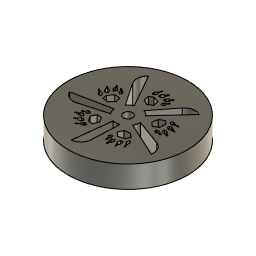
Mouse wheel (Autodesk Fusion 360 design; units mm, degrees)
Autodesk Fusion 360 part; units mm, degrees
(part 1 of 2)
sketch "Sketch1" plane through (0, 0, 0) normal (0, 0, 1) x (1, 0, 0)
  line L0 (-1.4367, 0.431) -> (1.4367, -0.431) construction
  arc A0 (-1.118, 1) -> (1.118, 1) centre (0, 0) ccw
  line L1 (-1.118, 1) -> (1.118, 1)
  line L2 (1.4367, 0.431) -> (-1.4367, -0.431) construction
  circle A1 centre (0, 0) radius 19
  dimension "d1" = 3
  dimension "d2" = 38
  constraint coincident A0.centre A1.centre
  constraint coincident L0 A0.centre
  constraint coincident A0 L2.end
  constraint coincident A0 L0.start
  constraint coincident A0 L0.end
  constraint coincident A0 L2.start
  constraint concentric A0 A1
  measures "d1" diameter of A0
  measures "d2" diameter of A1
extrude "Extrude1" add sketch "Sketch1" against normal blind 7 contours A0 L1 | A1
sketch "Sketch2" plane through (0, 0, 0) normal (0, 0, 1) x (-1, 0, 0)
  circle A0 centre (0, 0) radius 19
  circle A1 centre (0, 0) radius 3.5
  circle A2 centre (0, 0) radius 14
  dimension "d6" = 7
  dimension "d7" = 5
  constraint concentric A1 A2
  measures "d6" diameter of A1
  measures "d7" distance of A0 A2
sketch "Sketch3" plane through (0, 0, 0) normal (0, 0, 1) x (-1, 0, 0)
  line L0 (1.4245, 3.197) -> (4.8033, 7.8695)
  line L1 (4.8033, 7.8695) -> (-0.831, 15.5019)
  line L2 (-1.4884, 3.1677) -> (1.812, 7.535)
  line L3 (1.812, 7.535) -> (-5.6083, 14.6274)
  line L4 (-5.6083, 14.6274) -> (-0.831, 15.5019)
  line L5 (-1.4884, 3.1677) -> (-0.63, 3.41)
  line L6 (-0.63, 3.41) -> (1.4245, 3.197)
  line L7 (-3.4727, -0.4367) -> (-6.6062, 4.0518)
  line L8 (-2.6003, 2.3427) -> (-6, 7)
  line L9 (-6, 7) -> (-15, 4)
  line L10 (-6.6062, 4.0518) -> (-15.6446, -0.8137)
  line L11 (-15.6446, -0.8137) -> (-15, 4)
  line L12 (-3.4378, 0.4546) -> (-2.6003, 2.3427)
  line L13 (-3.4727, -0.4367) -> (-3.4378, 0.4546)
  line L14 (-0.6578, -3.4376) -> (-5.8949, -5.0308)
  line L15 (-3.0316, -1.7491) -> (-8.5115, -3.5432)
  line L16 (-8.5115, -3.5432) -> (-8.4395, -13.0298)
  line L17 (-5.8949, -5.0308) -> (-4.0605, -15.1303)
  line L18 (-4.0605, -15.1303) -> (-8.4395, -13.0298)
  line L19 (-1.4947, -3.1291) -> (-3.0316, -1.7491)
  line L20 (-0.6578, -3.4376) -> (-1.4947, -3.1291)
  line L21 (3.0661, -1.6879) -> (2.963, -7.161)
  line L22 (0.7267, -3.4237) -> (0.7396, -9.1898)
  line L23 (0.7396, -9.1898) -> (9.7841, -12.0528)
  line L24 (2.963, -7.161) -> (13.135, -8.5373)
  line L25 (13.135, -8.5373) -> (9.7841, -12.0528)
  line L26 (2.514, -2.3884) -> (0.7267, -3.4237)
  line L27 (3.0661, -1.6879) -> (2.514, -2.3884)
  line L28 (2.5528, 2.3945) -> (7.7261, 0.6051)
  line L29 (3.4807, -0.3669) -> (8.9686, -2.1364)
  line L30 (8.9686, -2.1364) -> (14.4864, 5.5807)
  line L31 (7.7261, 0.6051) -> (12.1784, 9.854)
  line L32 (12.1784, 9.854) -> (14.4864, 5.5807)
  line L33 (3.0484, 1.6529) -> (3.4807, -0.3669)
  line L34 (2.5528, 2.3945) -> (3.0484, 1.6529)
  circle A0 centre (0, 0) radius 19
  dimension "d11" = 360
sketch "Sketch4" plane through (0, 0, 0) normal (0, 0, 1) x (-1, 0, 0)
  circle A0 centre (0, 0) radius 19
  circle A1 centre (0, 0) radius 1.45
  dimension "d30" = 2.9
  constraint coincident A0.centre A1.centre
  measures "d30" diameter of A1
sketch "Sketch6" plane through (0, 0, 0) normal (0, 0, 1) x (-1, 0, 0)
  circle A0 centre (0, 0) radius 19
sketch "Sketch7" plane through (0, 0, 0) normal (0, 0, 1) x (-1, 0, 0)
  line L0 (0, -6) -> (1.6404, -6.8063)
  line L1 (1.6404, -6.8063) -> (2, -8.5)
  line L2 (2, -8.5) -> (0.8202, -9.1077)
  line L3 (0.8202, -9.1077) -> (-1, -8.5)
  line L4 (-1, -8.5) -> (-1.357, -6.8189)
  line L5 (-1.357, -6.8189) -> (0, -6)
  line L6 (1.9455, -9.6677) -> (2.2324, -10.2247)
  line L7 (2.2324, -10.2247) -> (2.0889, -10.6544)
  line L8 (2.0889, -10.6544) -> (1.4101, -11.4226)
  line L9 (1.4101, -11.4226) -> (1.2014, -10.4396)
  line L10 (1.2014, -10.4396) -> (1.3057, -10.127)
  line L11 (1.3057, -10.127) -> (1.9455, -9.6677)
  line L12 (0.4215, -10.1911) -> (0.4215, -10.8376)
  line L13 (0.4215, -10.8376) -> (-0.1481, -11.4996)
  line L14 (-0.1481, -11.4996) -> (-0.7484, -11.4996)
  line L15 (-0.7484, -11.4996) -> (-0.7484, -10.5143)
  line L16 (-0.7484, -10.5143) -> (-0.1481, -10.0371)
  line L17 (-0.1481, -10.0371) -> (0.4215, -10.1911)
  line L18 (-1.3334, -9.8678) -> (-1.5082, -10.5143)
  line L19 (-1.5082, -10.5143) -> (-2.1168, -10.9982)
  line L20 (-2.1168, -10.9982) -> (-2.5, -10.9982)
  line L21 (-2.5, -10.9982) -> (-2.7496, -10.5143)
  line L22 (-2.7496, -10.5143) -> (-2.3084, -9.7293)
  line L23 (-2.3084, -9.7293) -> (-1.3334, -9.8678)
  line L24 (-2.3084, -9.1135) -> (-3.0575, -9.2674)
  line L25 (-3.0575, -9.2674) -> (-3.1911, -8.6176)
  line L26 (-2.3084, -9.1135) -> (-2.1907, -8.2851)
  line L27 (-2.1907, -8.2851) -> (-2.8295, -8.1943)
  line L28 (-2.8295, -8.1943) -> (-3.1911, -8.6176)
  line L29 (1.4529, -11.869) -> (1.1049, -12.2764)
  line L30 (1.1049, -12.2764) -> (1.1894, -11.6818)
  line L31 (1.1894, -11.6818) -> (1.4101, -11.6349)
  line L32 (1.4101, -11.6349) -> (1.4529, -11.869)
  line L33 (-0.5833, -11.869) -> (-0.9521, -12.3007)
  line L34 (-0.9521, -12.3007) -> (-0.9521, -11.7519)
  line L35 (-0.9521, -11.7519) -> (-0.7677, -11.7519)
  line L36 (-0.7677, -11.7519) -> (-0.5833, -11.869)
  line L37 (-2.6562, -11.3012) -> (-3.1065, -11.6591)
  line L38 (-3.1065, -11.6591) -> (-2.9735, -11.007)
  line L39 (-2.9735, -11.007) -> (-2.7469, -11.007)
  line L40 (-2.7469, -11.007) -> (-2.6562, -11.3012)
  line L41 (-3.04, -9.5445) -> (-3.04, -9.7825)
  line L42 (-3.04, -9.7825) -> (-3.4222, -10.0863)
  line L43 (-3.4222, -10.0863) -> (-3.4222, -9.6635)
  line L44 (-3.4222, -9.6635) -> (-3.2311, -9.5116)
  line L45 (-3.2311, -9.5116) -> (-3.04, -9.5445)
  line L46 (11.2993, -2.1887) -> (10.2999, -2.0834)
  line L47 (10.7785, -1.3057) -> (11.2993, -2.1887)
  line L48 (10.4141, -1.0365) -> (10.7785, -1.3057)
  line L49 (9.7957, -1.1372) -> (10.4141, -1.0365)
  line L50 (10.0348, -1.8876) -> (9.7957, -1.1372)
  line L51 (10.2999, -2.0834) -> (10.0348, -1.8876)
  line L52 (8.702, -0.7245) -> (8.9154, -2.0344)
  line L53 (6.9801, -0.5432) -> (8.702, -0.7245)
  line L54 (5.7063, -1.8541) -> (6.9801, -0.5432)
  line L55 (6.0658, -3.3977) -> (5.7063, -1.8541)
  line L56 (7.775, -3.5777) -> (6.0658, -3.3977)
  line L57 (8.9154, -2.0344) -> (7.775, -3.5777)
  line L58 (7.2026, -4.6437) -> (6.9189, -5.2232)
  line L59 (7.9541, -5.0117) -> (7.2026, -4.6437)
  line L60 (7.9541, -5.0117) -> (7.869, -5.7717)
  line L61 (7.869, -5.7717) -> (7.2097, -5.6979)
  line L62 (6.9189, -5.2232) -> (7.2097, -5.6979)
  line L63 (10.4374, -2.9482) -> (10.891, -3.6944)
  line L64 (9.8225, -2.7484) -> (10.4374, -2.9482)
  line L65 (9.5001, -3.2425) -> (9.8225, -2.7484)
  line L66 (9.7685, -3.9609) -> (9.5001, -3.2425)
  line L67 (10.7054, -4.2654) -> (9.7685, -3.9609)
  line L68 (10.891, -3.6944) -> (10.7054, -4.2654)
  line L69 (12.0169, -2.7428) -> (11.4775, -2.4787)
  line L70 (11.7371, -2.286) -> (12.0169, -2.7428)
  line L71 (11.5012, -2.2543) -> (11.7371, -2.286)
  line L72 (11.4775, -2.4787) -> (11.5012, -2.2543)
  line L73 (11.1078, -4.2225) -> (11.4045, -4.7067)
  line L74 (10.9395, -4.3617) -> (11.1078, -4.2225)
  line L75 (10.8825, -4.5371) -> (10.9395, -4.3617)
  line L76 (11.4045, -4.7067) -> (10.8825, -4.5371)
  line L77 (9.5337, -4.6835) -> (9.8057, -5.4118)
  line L78 (8.9728, -4.3175) -> (9.5337, -4.6835)
  line L79 (8.5397, -5.2019) -> (8.9728, -4.3175)
  line L80 (9.1501, -5.8642) -> (8.5397, -5.2019)
  line L81 (9.6873, -5.7763) -> (9.1501, -5.8642)
  line L82 (9.8057, -5.4118) -> (9.6873, -5.7763)
  line L83 (9.9272, -6.0184) -> (10.1285, -6.5574)
  line L84 (9.6194, -6.0137) -> (9.9272, -6.0184)
  line L85 (10.1285, -6.5574) -> (9.5494, -6.2293)
  line L86 (9.5494, -6.2293) -> (9.6194, -6.0137)
  line L87 (8.3643, -5.9142) -> (8.5351, -6.3715)
  line L88 (8.5351, -6.3715) -> (8.133, -6.2409)
  line L89 (8.133, -6.2409) -> (8.0476, -6.0122)
  line L90 (8.0476, -6.0122) -> (8.138, -5.8407)
  line L91 (8.138, -5.8407) -> (8.3643, -5.9142)
  line L92 (5.5732, 10.0699) -> (5.1643, 9.1519)
  line L93 (4.5725, 9.8475) -> (5.5732, 10.0699)
  line L94 (4.2039, 9.5842) -> (4.5725, 9.8475)
  line L95 (4.1086, 8.9648) -> (4.2039, 9.5842)
  line L96 (4.8961, 8.9604) -> (4.1086, 8.9648)
  line L97 (5.1643, 9.1519) -> (4.8961, 8.9604)
  line L98 (3.3781, 8.0522) -> (4.6898, 7.8504)
  line L99 (2.6736, 6.4706) -> (3.3781, 8.0522)
  line L100 (3.5267, 4.8541) -> (2.6736, 6.4706)
  line L101 (5.1059, 4.719) -> (3.5267, 4.8541)
  line L102 (5.8052, 6.2889) -> (5.1059, 4.719)
  line L103 (4.6898, 7.8504) -> (5.8052, 6.2889)
  line L104 (6.6422, 5.4151) -> (7.1056, 4.9662)
  line L105 (7.2243, 6.0161) -> (6.6422, 5.4151)
  line L106 (7.2243, 6.0161) -> (7.9209, 5.7004)
  line L107 (7.9209, 5.7004) -> (7.6469, 5.0961)
  line L108 (7.1056, 4.9662) -> (7.6469, 5.0961)
  line L109 (6.0292, 9.0156) -> (6.8791, 9.2163)
  line L110 (5.6492, 8.4925) -> (6.0292, 9.0156)
  line L111 (6.0195, 8.0332) -> (5.6492, 8.4925)
  line L112 (6.7857, 8.0664) -> (6.0195, 8.0332)
  line L113 (7.3648, 8.8634) -> (6.7857, 8.0664)
  line L114 (6.8791, 9.2163) -> (7.3648, 8.8634)
  line L115 (6.322, 10.5812) -> (5.9041, 10.1498)
  line L116 (5.801, 10.4562) -> (6.322, 10.5812)
  line L117 (5.698, 10.2417) -> (5.801, 10.4562)
  line L118 (5.9041, 10.1498) -> (5.698, 10.2417)
  line L119 (7.4483, 9.2594) -> (8.0005, 9.3919)
  line L120 (7.5287, 9.0563) -> (7.4483, 9.2594)
  line L121 (7.6779, 8.9479) -> (7.5287, 9.0563)
  line L122 (8.0005, 9.3919) -> (7.6779, 8.9479)
  line L123 (7.4003, 7.6198) -> (8.1771, 7.6535)
  line L124 (6.8789, 7.1995) -> (7.4003, 7.6198)
  line L125 (7.5863, 6.5143) -> (6.8789, 7.1995)
  line L126 (8.4047, 6.8901) -> (7.5863, 6.5143)
  line L127 (8.4871, 7.4282) -> (8.4047, 6.8901)
  line L128 (8.1771, 7.6535) -> (8.4871, 7.4282)
  line L129 (8.7916, 7.5816) -> (9.3663, 7.6065)
  line L130 (8.692, 7.2903) -> (8.7916, 7.5816)
  line L131 (9.3663, 7.6065) -> (8.8753, 7.157)
  line L132 (8.8753, 7.157) -> (8.692, 7.2903)
  line L133 (8.2095, 6.1273) -> (8.6972, 6.1485)
  line L134 (8.6972, 6.1485) -> (8.4487, 5.8064)
  line L135 (8.4487, 5.8064) -> (8.2048, 5.7959)
  line L136 (8.2048, 5.7959) -> (8.0696, 5.9348)
  line L137 (8.0696, 5.9348) -> (8.2095, 6.1273)
  line L138 (-7.8548, 8.4122) -> (-7.1081, 7.7396)
  line L139 (-7.9525, 7.3918) -> (-7.8548, 8.4122)
  line L140 (-7.816, 6.9598) -> (-7.9525, 7.3918)
  line L141 (-7.2564, 6.6778) -> (-7.816, 6.9598)
  line L142 (-7.0089, 7.4254) -> (-7.2564, 6.6778)
  line L143 (-7.1081, 7.7396) -> (-7.0089, 7.4254)
  line L144 (-6.6142, 5.7011) -> (-6.0169, 6.8862)
  line L145 (-5.3277, 4.5422) -> (-6.6142, 5.7011)
  line L146 (-3.5267, 4.8541) -> (-5.3277, 4.5422)
  line L147 (-2.9103, 6.3142) -> (-3.5267, 4.8541)
  line L148 (-4.1872, 7.4644) -> (-2.9103, 6.3142)
  line L149 (-6.0169, 6.8862) -> (-4.1872, 7.4644)
  line L150 (-3.0976, 7.9904) -> (-2.5274, 8.2925)
  line L151 (-3.4892, 8.7298) -> (-3.0976, 7.9904)
  line L152 (-3.4892, 8.7298) -> (-2.9737, 9.2947)
  line L153 (-2.9737, 9.2947) -> (-2.4836, 8.8474)
  line L154 (-2.5274, 8.2925) -> (-2.4836, 8.8474)
  line L155 (-6.7112, 8.5201) -> (-6.6395, 9.3904)
  line L156 (-6.3312, 7.997) -> (-6.7112, 8.5201)
  line L157 (-5.7799, 8.2073) -> (-6.3312, 7.997)
  line L158 (-5.5747, 8.9462) -> (-5.7799, 8.2073)
  line L159 (-6.1538, 9.7433) -> (-5.5747, 8.9462)
  line L160 (-6.6395, 9.3904) -> (-6.1538, 9.7433)
  line L161 (-8.1097, 9.2824) -> (-7.8286, 8.7516)
  line L162 (-8.1518, 8.7483) -> (-8.1097, 9.2824)
  line L163 (-7.9796, 8.584) -> (-8.1518, 8.7483)
  line L164 (-7.8286, 8.7516) -> (-7.9796, 8.584)
  line L165 (-6.5045, 9.9451) -> (-6.4599, 10.5111)
  line L166 (-6.2865, 9.9588) -> (-6.5045, 9.9451)
  line L167 (-6.1373, 10.0672) -> (-6.2865, 9.9588)
  line L168 (-6.4599, 10.5111) -> (-6.1373, 10.0672)
  line L169 (-4.9601, 9.3928) -> (-4.752, 10.1419)
  line L170 (-4.7214, 8.767) -> (-4.9601, 9.3928)
  line L171 (-3.8512, 9.228) -> (-4.7214, 8.767)
  line L172 (-3.9557, 10.1225) -> (-3.8512, 9.228)
  line L173 (-4.442, 10.3672) -> (-3.9557, 10.1225)
  line L174 (-4.752, 10.1419) -> (-4.442, 10.3672)
  line L175 (-4.4938, 10.7041) -> (-4.3398, 11.2584)
  line L176 (-4.2475, 10.5194) -> (-4.4938, 10.7041)
  line L177 (-4.3398, 11.2584) -> (-4.0641, 10.6526)
  line L178 (-4.0641, 10.6526) -> (-4.2475, 10.5194)
  line L179 (-3.2906, 9.7011) -> (-3.16, 10.1715)
  line L180 (-3.16, 10.1715) -> (-2.9115, 9.8295)
  line L181 (-2.9115, 9.8295) -> (-2.9768, 9.5943)
  line L182 (-2.9768, 9.5943) -> (-3.1507, 9.5086)
  line L183 (-3.1507, 9.5086) -> (-3.2906, 9.7011)
  line L184 (-10.4278, -4.8709) -> (-9.5574, -4.3686)
  line L185 (-9.4874, -5.2791) -> (-10.4278, -4.8709)
  line L186 (-9.0344, -5.2828) -> (-9.4874, -5.2791)
  line L187 (-8.5933, -4.8377) -> (-9.0344, -5.2828)
  line L188 (-9.2278, -4.3712) -> (-8.5933, -4.8377)
  line L189 (-9.5574, -4.3686) -> (-9.2278, -4.3712)
  line L190 (-7.4659, -4.5288) -> (-8.4085, -3.5945)
  line L191 (-5.9663, -3.6633) -> (-7.4659, -4.5288)
  line L192 (-5.7063, -1.8541) -> (-5.9663, -3.6633)
  line L193 (-6.9045, -0.8166) -> (-5.7063, -1.8541)
  line L194 (-8.393, -1.6756) -> (-6.9045, -0.8166)
  line L195 (-8.4085, -3.5945) -> (-8.393, -1.6756)
  line L196 (-8.5566, -0.4768) -> (-8.6676, 0.1588)
  line L197 (-9.3808, -0.6208) -> (-8.5566, -0.4768)
  line L198 (-9.3808, -0.6208) -> (-9.7587, 0.0441)
  line L199 (-9.7587, 0.0441) -> (-9.1819, 0.3719)
  line L200 (-8.6676, 0.1588) -> (-9.1819, 0.3719)
  line L201 (-10.1769, -3.7499) -> (-10.9825, -3.4127)
  line L202 (-9.562, -3.5501) -> (-10.1769, -3.7499)
  line L203 (-9.5916, -2.9608) -> (-9.562, -3.5501)
  line L204 (-10.231, -2.5373) -> (-9.5916, -2.9608)
  line L205 (-11.168, -2.8417) -> (-10.231, -2.5373)
  line L206 (-10.9825, -3.4127) -> (-11.168, -2.8417)
  line L207 (-11.3341, -4.8444) -> (-10.7425, -4.741)
  line L208 (-10.8391, -5.0495) -> (-11.3341, -4.8444)
  line L209 (-10.6297, -4.9365) -> (-10.8391, -5.0495)
  line L210 (-10.7425, -4.741) -> (-10.6297, -4.9365)
  line L211 (-11.4683, -3.113) -> (-11.9929, -2.8956)
  line L212 (-11.414, -2.9014) -> (-11.4683, -3.113)
  line L213 (-11.471, -2.726) -> (-11.414, -2.9014)
  line L214 (-11.9929, -2.8956) -> (-11.471, -2.726)
  line L215 (-10.4658, -1.8148) -> (-11.114, -1.3854)
  line L216 (-9.7969, -1.7812) -> (-10.4658, -1.8148)
  line L217 (-9.9664, -0.8111) -> (-9.7969, -1.7812)
  line L218 (-10.8494, -0.634) -> (-9.9664, -0.8111)
  line L219 (-11.2324, -1.021) -> (-10.8494, -0.634)
  line L220 (-11.114, -1.3854) -> (-11.2324, -1.021)
  line L221 (-11.5688, -0.9661) -> (-12.0485, -0.6484)
  line L222 (-11.3171, -0.7889) -> (-11.5688, -0.9661)
  line L223 (-12.0485, -0.6484) -> (-11.3871, -0.5734)
  line L224 (-11.3871, -0.5734) -> (-11.3171, -0.7889)
  line L225 (-10.2432, -0.1317) -> (-10.6502, 0.1379)
  line L226 (-10.6502, 0.1379) -> (-10.2481, 0.2685)
  line L227 (-10.2481, 0.2685) -> (-10.0446, 0.1337)
  line L228 (-10.0446, 0.1337) -> (-10.0168, -0.0582)
  line L229 (-10.0168, -0.0582) -> (-10.2432, -0.1317)
  dimension "d34" = 360
  constraint parallel L1 L4
  constraint perpendicular L2 L6
  constraint perpendicular L3 L7
  constraint parallel L4 L9
  constraint perpendicular L3 L10
  constraint vertical L12
  constraint horizontal L14
  constraint perpendicular L14 L15
  constraint perpendicular L17 L18
  constraint parallel L16 L19
  constraint perpendicular L12 L20
  constraint perpendicular L24 L25
  constraint perpendicular L23 L26
  constraint perpendicular L26 L27
  constraint parallel L28 L29
  constraint perpendicular L23 L30
  constraint perpendicular L9 L31
  constraint parallel L29 L33
  constraint vertical L34
  constraint perpendicular L34 L35
  constraint parallel L16 L37
  constraint perpendicular L39 L41
  constraint parallel L37 L42
  constraint perpendicular L39 L43
  constraint parallel L37 L44
extrude "Extrude9" cut sketch "Sketch7" against normal blind 17
sketch "Sketch8" plane through (0, 0, 0) normal (0, 0, 1) x (-1, 0, 0)
  line L0 (-3.1065, -11.6591) -> (-2.9735, -11.007)
  line L1 (-2.9735, -11.007) -> (-2.7469, -11.007)
  line L2 (-2.7469, -11.007) -> (-2.6562, -11.3012)
  line L3 (-2.6562, -11.3012) -> (-3.1065, -11.6591)
  line L4 (-11.5688, -0.9661) -> (-12.0485, -0.6484)
  line L5 (-12.0485, -0.6484) -> (-11.3871, -0.5734)
  line L6 (-11.3871, -0.5734) -> (-11.3171, -0.7889)
  line L7 (-11.3171, -0.7889) -> (-11.5688, -0.9661)
  line L8 (-4.4938, 10.7041) -> (-4.3398, 11.2584)
  line L9 (-4.3398, 11.2584) -> (-4.0641, 10.6526)
  line L10 (-4.0641, 10.6526) -> (-4.2475, 10.5194)
  line L11 (-4.2475, 10.5194) -> (-4.4938, 10.7041)
  line L12 (8.7916, 7.5816) -> (9.3663, 7.6065)
  line L13 (9.3663, 7.6065) -> (8.8753, 7.157)
  line L14 (8.8753, 7.157) -> (8.692, 7.2903)
  line L15 (8.692, 7.2903) -> (8.7916, 7.5816)
  line L16 (9.9272, -6.0184) -> (10.1285, -6.5574)
  line L17 (10.1285, -6.5574) -> (9.5494, -6.2293)
  line L18 (9.5494, -6.2293) -> (9.6194, -6.0137)
  line L19 (9.6194, -6.0137) -> (9.9272, -6.0184)
  line L20 (-2.5, -10.9982) -> (-2.7496, -10.5143)
  line L21 (-2.7496, -10.5143) -> (-2.3084, -9.7293)
  line L22 (-2.3084, -9.7293) -> (-1.3334, -9.8678)
  line L23 (-1.3334, -9.8678) -> (-1.5082, -10.5143)
  line L24 (-1.5082, -10.5143) -> (-2.1168, -10.9982)
  line L25 (-2.1168, -10.9982) -> (-2.5, -10.9982)
  line L26 (-9.7969, -1.7812) -> (-10.4658, -1.8148)
  line L27 (-10.4658, -1.8148) -> (-11.114, -1.3854)
  line L28 (-11.114, -1.3854) -> (-11.2324, -1.021)
  line L29 (-11.2324, -1.021) -> (-10.8494, -0.634)
  line L30 (-10.8494, -0.634) -> (-9.9664, -0.8111)
  line L31 (-9.9664, -0.8111) -> (-9.7969, -1.7812)
  line L32 (-4.7214, 8.767) -> (-4.9601, 9.3928)
  line L33 (-4.9601, 9.3928) -> (-4.752, 10.1419)
  line L34 (-4.752, 10.1419) -> (-4.442, 10.3672)
  line L35 (-4.442, 10.3672) -> (-3.9557, 10.1225)
  line L36 (-3.9557, 10.1225) -> (-3.8512, 9.228)
  line L37 (-3.8512, 9.228) -> (-4.7214, 8.767)
  line L38 (6.8789, 7.1995) -> (7.4003, 7.6198)
  line L39 (7.4003, 7.6198) -> (8.1771, 7.6535)
  line L40 (8.1771, 7.6535) -> (8.4871, 7.4282)
  line L41 (8.4871, 7.4282) -> (8.4047, 6.8901)
  line L42 (8.4047, 6.8901) -> (7.5863, 6.5143)
  line L43 (7.5863, 6.5143) -> (6.8789, 7.1995)
  line L44 (8.9728, -4.3175) -> (9.5337, -4.6835)
  line L45 (9.5337, -4.6835) -> (9.8057, -5.4118)
  line L46 (9.8057, -5.4118) -> (9.6873, -5.7763)
  line L47 (9.6873, -5.7763) -> (9.1501, -5.8642)
  line L48 (9.1501, -5.8642) -> (8.5397, -5.2019)
  line L49 (8.5397, -5.2019) -> (8.9728, -4.3175)
  line L50 (-5.9663, -3.6633) -> (-7.4659, -4.5288)
  line L51 (-7.4659, -4.5288) -> (-8.4085, -3.5945)
  line L52 (-8.4085, -3.5945) -> (-8.393, -1.6756)
  line L53 (-8.393, -1.6756) -> (-6.9045, -0.8166)
  line L54 (-6.9045, -0.8166) -> (-5.7063, -1.8541)
  line L55 (-5.7063, -1.8541) -> (-5.9663, -3.6633)
  line L56 (-5.3277, 4.5422) -> (-6.6142, 5.7011)
  line L57 (-6.6142, 5.7011) -> (-6.0169, 6.8862)
  line L58 (-6.0169, 6.8862) -> (-4.1872, 7.4644)
  line L59 (-4.1872, 7.4644) -> (-2.9103, 6.3142)
  line L60 (-2.9103, 6.3142) -> (-3.5267, 4.8541)
  line L61 (-3.5267, 4.8541) -> (-5.3277, 4.5422)
  line L62 (6.9189, -5.2232) -> (7.2026, -4.6437)
  line L63 (7.2026, -4.6437) -> (7.9541, -5.0117)
  line L64 (7.9541, -5.0117) -> (7.869, -5.7717)
  line L65 (7.869, -5.7717) -> (7.2097, -5.6979)
  line L66 (7.2097, -5.6979) -> (6.9189, -5.2232)
  line L67 (7.1056, 4.9662) -> (6.6422, 5.4151)
  line L68 (6.6422, 5.4151) -> (7.2243, 6.0161)
  line L69 (7.2243, 6.0161) -> (7.9209, 5.7004)
  line L70 (7.9209, 5.7004) -> (7.6469, 5.0961)
  line L71 (7.6469, 5.0961) -> (7.1056, 4.9662)
  line L72 (-2.5274, 8.2925) -> (-3.0976, 7.9904)
  line L73 (-3.0976, 7.9904) -> (-3.4892, 8.7298)
  line L74 (-3.4892, 8.7298) -> (-2.9737, 9.2947)
  line L75 (-2.9737, 9.2947) -> (-2.4836, 8.8474)
  line L76 (-2.4836, 8.8474) -> (-2.5274, 8.2925)
  line L77 (-8.6676, 0.1588) -> (-8.5566, -0.4768)
  line L78 (-8.5566, -0.4768) -> (-9.3808, -0.6208)
  line L79 (-9.3808, -0.6208) -> (-9.7587, 0.0441)
  line L80 (-9.7587, 0.0441) -> (-9.1819, 0.3719)
  line L81 (-9.1819, 0.3719) -> (-8.6676, 0.1588)
  line L82 (-2.8295, -8.1943) -> (-2.1907, -8.2851)
  line L83 (-2.1907, -8.2851) -> (-2.3084, -9.1135)
  line L84 (-2.3084, -9.1135) -> (-3.0575, -9.2674)
  line L85 (-3.0575, -9.2674) -> (-3.1911, -8.6176)
  line L86 (-3.1911, -8.6176) -> (-2.8295, -8.1943)
  line L87 (8.133, -6.2409) -> (8.0476, -6.0122)
  line L88 (8.0476, -6.0122) -> (8.138, -5.8407)
  line L89 (8.138, -5.8407) -> (8.3643, -5.9142)
  line L90 (8.3643, -5.9142) -> (8.5351, -6.3715)
  line L91 (8.5351, -6.3715) -> (8.133, -6.2409)
  line L92 (8.4487, 5.8064) -> (8.2048, 5.7959)
  line L93 (8.2048, 5.7959) -> (8.0696, 5.9348)
  line L94 (8.0696, 5.9348) -> (8.2095, 6.1273)
  line L95 (8.2095, 6.1273) -> (8.6972, 6.1485)
  line L96 (8.6972, 6.1485) -> (8.4487, 5.8064)
  line L97 (-2.9115, 9.8295) -> (-2.9768, 9.5943)
  line L98 (-2.9768, 9.5943) -> (-3.1507, 9.5086)
  line L99 (-3.1507, 9.5086) -> (-3.2906, 9.7011)
  line L100 (-3.2906, 9.7011) -> (-3.16, 10.1715)
  line L101 (-3.16, 10.1715) -> (-2.9115, 9.8295)
  line L102 (-10.2481, 0.2685) -> (-10.0446, 0.1337)
  line L103 (-10.0446, 0.1337) -> (-10.0168, -0.0582)
  line L104 (-10.0168, -0.0582) -> (-10.2432, -0.1317)
  line L105 (-10.2432, -0.1317) -> (-10.6502, 0.1379)
  line L106 (-10.6502, 0.1379) -> (-10.2481, 0.2685)
  line L107 (-3.4222, -10.0863) -> (-3.4222, -9.6635)
  line L108 (-3.4222, -9.6635) -> (-3.2311, -9.5116)
  line L109 (-3.2311, -9.5116) -> (-3.04, -9.5445)
  line L110 (-3.04, -9.5445) -> (-3.04, -9.7825)
  line L111 (-3.04, -9.7825) -> (-3.4222, -10.0863)
  line L112 (-0.9521, -12.3007) -> (-0.9521, -11.7519)
  line L113 (-0.9521, -11.7519) -> (-0.7677, -11.7519)
  line L114 (-0.7677, -11.7519) -> (-0.5833, -11.869)
  line L115 (-0.5833, -11.869) -> (-0.9521, -12.3007)
  line L116 (-11.414, -2.9014) -> (-11.4683, -3.113)
  line L117 (-11.4683, -3.113) -> (-11.9929, -2.8956)
  line L118 (-11.9929, -2.8956) -> (-11.471, -2.726)
  line L119 (-11.471, -2.726) -> (-11.414, -2.9014)
  line L120 (-6.2865, 9.9588) -> (-6.5045, 9.9451)
  line L121 (-6.5045, 9.9451) -> (-6.4599, 10.5111)
  line L122 (-6.4599, 10.5111) -> (-6.1373, 10.0672)
  line L123 (-6.1373, 10.0672) -> (-6.2865, 9.9588)
  line L124 (7.5287, 9.0563) -> (7.4483, 9.2594)
  line L125 (7.4483, 9.2594) -> (8.0005, 9.3919)
  line L126 (8.0005, 9.3919) -> (7.6779, 8.9479)
  line L127 (7.6779, 8.9479) -> (7.5287, 9.0563)
  line L128 (10.9395, -4.3617) -> (11.1078, -4.2225)
  line L129 (11.1078, -4.2225) -> (11.4045, -4.7067)
  line L130 (11.4045, -4.7067) -> (10.8825, -4.5371)
  line L131 (10.8825, -4.5371) -> (10.9395, -4.3617)
  line L132 (-0.7484, -11.4996) -> (-0.7484, -10.5143)
  line L133 (-0.7484, -10.5143) -> (-0.1481, -10.0371)
  line L134 (-0.1481, -10.0371) -> (0.4215, -10.1911)
  line L135 (0.4215, -10.1911) -> (0.4215, -10.8376)
  line L136 (0.4215, -10.8376) -> (-0.1481, -11.4996)
  line L137 (-0.1481, -11.4996) -> (-0.7484, -11.4996)
  line L138 (-9.562, -3.5501) -> (-10.1769, -3.7499)
  line L139 (-10.1769, -3.7499) -> (-10.9825, -3.4127)
  line L140 (-10.9825, -3.4127) -> (-11.168, -2.8417)
  line L141 (-11.168, -2.8417) -> (-10.231, -2.5373)
  line L142 (-10.231, -2.5373) -> (-9.5916, -2.9608)
  line L143 (-9.5916, -2.9608) -> (-9.562, -3.5501)
  line L144 (-6.3312, 7.997) -> (-6.7112, 8.5201)
  line L145 (-6.7112, 8.5201) -> (-6.6395, 9.3904)
  line L146 (-6.6395, 9.3904) -> (-6.1538, 9.7433)
  line L147 (-6.1538, 9.7433) -> (-5.5747, 8.9462)
  line L148 (-5.5747, 8.9462) -> (-5.7799, 8.2073)
  line L149 (-5.7799, 8.2073) -> (-6.3312, 7.997)
  line L150 (5.6492, 8.4925) -> (6.0292, 9.0156)
  line L151 (6.0292, 9.0156) -> (6.8791, 9.2163)
  line L152 (6.8791, 9.2163) -> (7.3648, 8.8634)
  line L153 (7.3648, 8.8634) -> (6.7857, 8.0664)
  line L154 (6.7857, 8.0664) -> (6.0195, 8.0332)
  line L155 (6.0195, 8.0332) -> (5.6492, 8.4925)
  line L156 (9.8225, -2.7484) -> (10.4374, -2.9482)
  line L157 (10.4374, -2.9482) -> (10.891, -3.6944)
  line L158 (10.891, -3.6944) -> (10.7054, -4.2654)
  line L159 (10.7054, -4.2654) -> (9.7685, -3.9609)
  line L160 (9.7685, -3.9609) -> (9.5001, -3.2425)
  line L161 (9.5001, -3.2425) -> (9.8225, -2.7484)
  line L162 (0.8202, -9.1077) -> (-1, -8.5)
  line L163 (-1, -8.5) -> (-1.357, -6.8189)
  line L164 (-1.357, -6.8189) -> (0, -6)
  line L165 (0, -6) -> (1.6404, -6.8063)
  line L166 (1.6404, -6.8063) -> (2, -8.5)
  line L167 (2, -8.5) -> (0.8202, -9.1077)
  line L168 (2.6736, 6.4706) -> (3.3781, 8.0522)
  line L169 (3.3781, 8.0522) -> (4.6898, 7.8504)
  line L170 (4.6898, 7.8504) -> (5.8052, 6.2889)
  line L171 (5.8052, 6.2889) -> (5.1059, 4.719)
  line L172 (5.1059, 4.719) -> (3.5267, 4.8541)
  line L173 (3.5267, 4.8541) -> (2.6736, 6.4706)
  line L174 (6.9801, -0.5432) -> (8.702, -0.7245)
  line L175 (8.702, -0.7245) -> (8.9154, -2.0344)
  line L176 (8.9154, -2.0344) -> (7.775, -3.5777)
  line L177 (7.775, -3.5777) -> (6.0658, -3.3977)
  line L178 (6.0658, -3.3977) -> (5.7063, -1.8541)
  line L179 (5.7063, -1.8541) -> (6.9801, -0.5432)
  line L180 (10.7785, -1.3057) -> (11.2993, -2.1887)
  line L181 (11.2993, -2.1887) -> (10.2999, -2.0834)
  line L182 (10.2999, -2.0834) -> (10.0348, -1.8876)
  line L183 (10.0348, -1.8876) -> (9.7957, -1.1372)
  line L184 (9.7957, -1.1372) -> (10.4141, -1.0365)
  line L185 (10.4141, -1.0365) -> (10.7785, -1.3057)
  line L186 (4.5725, 9.8475) -> (5.5732, 10.0699)
  line L187 (5.5732, 10.0699) -> (5.1643, 9.1519)
  line L188 (5.1643, 9.1519) -> (4.8961, 8.9604)
  line L189 (4.8961, 8.9604) -> (4.1086, 8.9648)
  line L190 (4.1086, 8.9648) -> (4.2039, 9.5842)
  line L191 (4.2039, 9.5842) -> (4.5725, 9.8475)
  line L192 (-7.9525, 7.3918) -> (-7.8548, 8.4122)
  line L193 (-7.8548, 8.4122) -> (-7.1081, 7.7396)
  line L194 (-7.1081, 7.7396) -> (-7.0089, 7.4254)
  line L195 (-7.0089, 7.4254) -> (-7.2564, 6.6778)
  line L196 (-7.2564, 6.6778) -> (-7.816, 6.9598)
  line L197 (-7.816, 6.9598) -> (-7.9525, 7.3918)
  line L198 (-9.4874, -5.2791) -> (-10.4278, -4.8709)
  line L199 (-10.4278, -4.8709) -> (-9.5574, -4.3686)
  line L200 (-9.5574, -4.3686) -> (-9.2278, -4.3712)
  line L201 (-9.2278, -4.3712) -> (-8.5933, -4.8377)
  line L202 (-8.5933, -4.8377) -> (-9.0344, -5.2828)
  line L203 (-9.0344, -5.2828) -> (-9.4874, -5.2791)
  line L204 (1.4101, -11.4226) -> (1.2014, -10.4396)
  line L205 (1.2014, -10.4396) -> (1.3057, -10.127)
  line L206 (1.3057, -10.127) -> (1.9455, -9.6677)
  line L207 (1.9455, -9.6677) -> (2.2324, -10.2247)
  line L208 (2.2324, -10.2247) -> (2.0889, -10.6544)
  line L209 (2.0889, -10.6544) -> (1.4101, -11.4226)
  line L210 (11.7371, -2.286) -> (12.0169, -2.7428)
  line L211 (12.0169, -2.7428) -> (11.4775, -2.4787)
  line L212 (11.4775, -2.4787) -> (11.5012, -2.2543)
  line L213 (11.5012, -2.2543) -> (11.7371, -2.286)
  line L214 (5.801, 10.4562) -> (6.322, 10.5812)
  line L215 (6.322, 10.5812) -> (5.9041, 10.1498)
  line L216 (5.9041, 10.1498) -> (5.698, 10.2417)
  line L217 (5.698, 10.2417) -> (5.801, 10.4562)
  line L218 (-8.1518, 8.7483) -> (-8.1097, 9.2824)
  line L219 (-8.1097, 9.2824) -> (-7.8286, 8.7516)
  line L220 (-7.8286, 8.7516) -> (-7.9796, 8.584)
  line L221 (-7.9796, 8.584) -> (-8.1518, 8.7483)
  line L222 (-10.8391, -5.0495) -> (-11.3341, -4.8444)
  line L223 (-11.3341, -4.8444) -> (-10.7425, -4.741)
  line L224 (-10.7425, -4.741) -> (-10.6297, -4.9365)
  line L225 (-10.6297, -4.9365) -> (-10.8391, -5.0495)
  line L226 (1.1049, -12.2764) -> (1.1894, -11.6818)
  line L227 (1.1894, -11.6818) -> (1.4101, -11.6349)
  line L228 (1.4101, -11.6349) -> (1.4529, -11.869)
  line L229 (1.4529, -11.869) -> (1.1049, -12.2764)
  circle A0 centre (0, 0) radius 19
  circle A1 centre (0, 0) radius 1.45
  circle A2 centre (0, 0) radius 16
  dimension "d37" = 2.9
  dimension "d38" = 3
  constraint concentric A0 A1
  constraint concentric A1 A2
  measures "d37" diameter of A1
  measures "d38" distance of A0 A2
extrude "Extrude10" cut sketch "Sketch8" against normal blind 15 contours A1
sketch "Sketch9" plane through (0, 0, 0) normal (0, 0, 1) x (-1, 0, 0)
  circle A0 centre (0, 0) radius 1.45
  line L0 (-3.1065, -11.6591) -> (-2.9735, -11.007)
  line L1 (-2.9735, -11.007) -> (-2.7469, -11.007)
  line L2 (-2.7469, -11.007) -> (-2.6562, -11.3012)
  line L3 (-2.6562, -11.3012) -> (-3.1065, -11.6591)
  line L4 (-11.5688, -0.9661) -> (-12.0485, -0.6484)
  line L5 (-12.0485, -0.6484) -> (-11.3871, -0.5734)
  line L6 (-11.3871, -0.5734) -> (-11.3171, -0.7889)
  line L7 (-11.3171, -0.7889) -> (-11.5688, -0.9661)
  line L8 (-4.4938, 10.7041) -> (-4.3398, 11.2584)
  line L9 (-4.3398, 11.2584) -> (-4.0641, 10.6526)
  line L10 (-4.0641, 10.6526) -> (-4.2475, 10.5194)
  line L11 (-4.2475, 10.5194) -> (-4.4938, 10.7041)
  line L12 (8.7916, 7.5816) -> (9.3663, 7.6065)
  line L13 (9.3663, 7.6065) -> (8.8753, 7.157)
  line L14 (8.8753, 7.157) -> (8.692, 7.2903)
  line L15 (8.692, 7.2903) -> (8.7916, 7.5816)
  line L16 (9.9272, -6.0184) -> (10.1285, -6.5574)
  line L17 (10.1285, -6.5574) -> (9.5494, -6.2293)
  line L18 (9.5494, -6.2293) -> (9.6194, -6.0137)
  line L19 (9.6194, -6.0137) -> (9.9272, -6.0184)
  line L20 (-2.5, -10.9982) -> (-2.7496, -10.5143)
  line L21 (-2.7496, -10.5143) -> (-2.3084, -9.7293)
  line L22 (-2.3084, -9.7293) -> (-1.3334, -9.8678)
  line L23 (-1.3334, -9.8678) -> (-1.5082, -10.5143)
  line L24 (-1.5082, -10.5143) -> (-2.1168, -10.9982)
  line L25 (-2.1168, -10.9982) -> (-2.5, -10.9982)
  line L26 (-9.7969, -1.7812) -> (-10.4658, -1.8148)
  line L27 (-10.4658, -1.8148) -> (-11.114, -1.3854)
  line L28 (-11.114, -1.3854) -> (-11.2324, -1.021)
  line L29 (-11.2324, -1.021) -> (-10.8494, -0.634)
  line L30 (-10.8494, -0.634) -> (-9.9664, -0.8111)
  line L31 (-9.9664, -0.8111) -> (-9.7969, -1.7812)
  line L32 (-4.7214, 8.767) -> (-4.9601, 9.3928)
  line L33 (-4.9601, 9.3928) -> (-4.752, 10.1419)
  line L34 (-4.752, 10.1419) -> (-4.442, 10.3672)
  line L35 (-4.442, 10.3672) -> (-3.9557, 10.1225)
  line L36 (-3.9557, 10.1225) -> (-3.8512, 9.228)
  line L37 (-3.8512, 9.228) -> (-4.7214, 8.767)
  line L38 (6.8789, 7.1995) -> (7.4003, 7.6198)
  line L39 (7.4003, 7.6198) -> (8.1771, 7.6535)
  line L40 (8.1771, 7.6535) -> (8.4871, 7.4282)
  line L41 (8.4871, 7.4282) -> (8.4047, 6.8901)
  line L42 (8.4047, 6.8901) -> (7.5863, 6.5143)
  line L43 (7.5863, 6.5143) -> (6.8789, 7.1995)
  line L44 (8.9728, -4.3175) -> (9.5337, -4.6835)
  line L45 (9.5337, -4.6835) -> (9.8057, -5.4118)
  line L46 (9.8057, -5.4118) -> (9.6873, -5.7763)
  line L47 (9.6873, -5.7763) -> (9.1501, -5.8642)
  line L48 (9.1501, -5.8642) -> (8.5397, -5.2019)
  line L49 (8.5397, -5.2019) -> (8.9728, -4.3175)
  line L50 (-5.9663, -3.6633) -> (-7.4659, -4.5288)
  line L51 (-7.4659, -4.5288) -> (-8.4085, -3.5945)
  line L52 (-8.4085, -3.5945) -> (-8.393, -1.6756)
  line L53 (-8.393, -1.6756) -> (-6.9045, -0.8166)
  line L54 (-6.9045, -0.8166) -> (-5.7063, -1.8541)
  line L55 (-5.7063, -1.8541) -> (-5.9663, -3.6633)
  line L56 (-5.3277, 4.5422) -> (-6.6142, 5.7011)
  line L57 (-6.6142, 5.7011) -> (-6.0169, 6.8862)
  line L58 (-6.0169, 6.8862) -> (-4.1872, 7.4644)
  line L59 (-4.1872, 7.4644) -> (-2.9103, 6.3142)
  line L60 (-2.9103, 6.3142) -> (-3.5267, 4.8541)
  line L61 (-3.5267, 4.8541) -> (-5.3277, 4.5422)
  line L62 (6.9189, -5.2232) -> (7.2026, -4.6437)
  line L63 (7.2026, -4.6437) -> (7.9541, -5.0117)
  line L64 (7.9541, -5.0117) -> (7.869, -5.7717)
  line L65 (7.869, -5.7717) -> (7.2097, -5.6979)
  line L66 (7.2097, -5.6979) -> (6.9189, -5.2232)
  line L67 (7.1056, 4.9662) -> (6.6422, 5.4151)
  line L68 (6.6422, 5.4151) -> (7.2243, 6.0161)
  line L69 (7.2243, 6.0161) -> (7.9209, 5.7004)
  line L70 (7.9209, 5.7004) -> (7.6469, 5.0961)
  line L71 (7.6469, 5.0961) -> (7.1056, 4.9662)
  line L72 (-2.5274, 8.2925) -> (-3.0976, 7.9904)
  line L73 (-3.0976, 7.9904) -> (-3.4892, 8.7298)
  line L74 (-3.4892, 8.7298) -> (-2.9737, 9.2947)
  line L75 (-2.9737, 9.2947) -> (-2.4836, 8.8474)
  line L76 (-2.4836, 8.8474) -> (-2.5274, 8.2925)
  line L77 (-8.6676, 0.1588) -> (-8.5566, -0.4768)
  line L78 (-8.5566, -0.4768) -> (-9.3808, -0.6208)
  line L79 (-9.3808, -0.6208) -> (-9.7587, 0.0441)
  line L80 (-9.7587, 0.0441) -> (-9.1819, 0.3719)
  line L81 (-9.1819, 0.3719) -> (-8.6676, 0.1588)
  line L82 (-2.8295, -8.1943) -> (-2.1907, -8.2851)
  line L83 (-2.1907, -8.2851) -> (-2.3084, -9.1135)
  line L84 (-2.3084, -9.1135) -> (-3.0575, -9.2674)
  line L85 (-3.0575, -9.2674) -> (-3.1911, -8.6176)
  line L86 (-3.1911, -8.6176) -> (-2.8295, -8.1943)
  line L87 (8.133, -6.2409) -> (8.0476, -6.0122)
  line L88 (8.0476, -6.0122) -> (8.138, -5.8407)
  line L89 (8.138, -5.8407) -> (8.3643, -5.9142)
  line L90 (8.3643, -5.9142) -> (8.5351, -6.3715)
  line L91 (8.5351, -6.3715) -> (8.133, -6.2409)
  line L92 (8.4487, 5.8064) -> (8.2048, 5.7959)
  line L93 (8.2048, 5.7959) -> (8.0696, 5.9348)
  line L94 (8.0696, 5.9348) -> (8.2095, 6.1273)
  line L95 (8.2095, 6.1273) -> (8.6972, 6.1485)
  line L96 (8.6972, 6.1485) -> (8.4487, 5.8064)
  line L97 (-2.9115, 9.8295) -> (-2.9768, 9.5943)
  line L98 (-2.9768, 9.5943) -> (-3.1507, 9.5086)
  line L99 (-3.1507, 9.5086) -> (-3.2906, 9.7011)
  line L100 (-3.2906, 9.7011) -> (-3.16, 10.1715)
  line L101 (-3.16, 10.1715) -> (-2.9115, 9.8295)
  line L102 (-10.2481, 0.2685) -> (-10.0446, 0.1337)
  line L103 (-10.0446, 0.1337) -> (-10.0168, -0.0582)
  line L104 (-10.0168, -0.0582) -> (-10.2432, -0.1317)
  line L105 (-10.2432, -0.1317) -> (-10.6502, 0.1379)
  line L106 (-10.6502, 0.1379) -> (-10.2481, 0.2685)
  line L107 (-3.4222, -10.0863) -> (-3.4222, -9.6635)
  line L108 (-3.4222, -9.6635) -> (-3.2311, -9.5116)
  line L109 (-3.2311, -9.5116) -> (-3.04, -9.5445)
  line L110 (-3.04, -9.5445) -> (-3.04, -9.7825)
  line L111 (-3.04, -9.7825) -> (-3.4222, -10.0863)
  line L112 (-0.9521, -12.3007) -> (-0.9521, -11.7519)
  line L113 (-0.9521, -11.7519) -> (-0.7677, -11.7519)
  line L114 (-0.7677, -11.7519) -> (-0.5833, -11.869)
  line L115 (-0.5833, -11.869) -> (-0.9521, -12.3007)
  line L116 (-11.414, -2.9014) -> (-11.4683, -3.113)
  line L117 (-11.4683, -3.113) -> (-11.9929, -2.8956)
  line L118 (-11.9929, -2.8956) -> (-11.471, -2.726)
  line L119 (-11.471, -2.726) -> (-11.414, -2.9014)
  line L120 (-6.2865, 9.9588) -> (-6.5045, 9.9451)
  line L121 (-6.5045, 9.9451) -> (-6.4599, 10.5111)
  line L122 (-6.4599, 10.5111) -> (-6.1373, 10.0672)
  line L123 (-6.1373, 10.0672) -> (-6.2865, 9.9588)
  line L124 (7.5287, 9.0563) -> (7.4483, 9.2594)
  line L125 (7.4483, 9.2594) -> (8.0005, 9.3919)
  line L126 (8.0005, 9.3919) -> (7.6779, 8.9479)
  line L127 (7.6779, 8.9479) -> (7.5287, 9.0563)
  line L128 (10.9395, -4.3617) -> (11.1078, -4.2225)
  line L129 (11.1078, -4.2225) -> (11.4045, -4.7067)
  line L130 (11.4045, -4.7067) -> (10.8825, -4.5371)
  line L131 (10.8825, -4.5371) -> (10.9395, -4.3617)
  line L132 (-0.7484, -11.4996) -> (-0.7484, -10.5143)
  line L133 (-0.7484, -10.5143) -> (-0.1481, -10.0371)
  line L134 (-0.1481, -10.0371) -> (0.4215, -10.1911)
  line L135 (0.4215, -10.1911) -> (0.4215, -10.8376)
  line L136 (0.4215, -10.8376) -> (-0.1481, -11.4996)
  line L137 (-0.1481, -11.4996) -> (-0.7484, -11.4996)
  line L138 (-9.562, -3.5501) -> (-10.1769, -3.7499)
  line L139 (-10.1769, -3.7499) -> (-10.9825, -3.4127)
  line L140 (-10.9825, -3.4127) -> (-11.168, -2.8417)
  line L141 (-11.168, -2.8417) -> (-10.231, -2.5373)
  line L142 (-10.231, -2.5373) -> (-9.5916, -2.9608)
  line L143 (-9.5916, -2.9608) -> (-9.562, -3.5501)
  line L144 (-6.3312, 7.997) -> (-6.7112, 8.5201)
  line L145 (-6.7112, 8.5201) -> (-6.6395, 9.3904)
  line L146 (-6.6395, 9.3904) -> (-6.1538, 9.7433)
  line L147 (-6.1538, 9.7433) -> (-5.5747, 8.9462)
  line L148 (-5.5747, 8.9462) -> (-5.7799, 8.2073)
  line L149 (-5.7799, 8.2073) -> (-6.3312, 7.997)
  line L150 (5.6492, 8.4925) -> (6.0292, 9.0156)
  line L151 (6.0292, 9.0156) -> (6.8791, 9.2163)
  line L152 (6.8791, 9.2163) -> (7.3648, 8.8634)
  line L153 (7.3648, 8.8634) -> (6.7857, 8.0664)
  line L154 (6.7857, 8.0664) -> (6.0195, 8.0332)
  line L155 (6.0195, 8.0332) -> (5.6492, 8.4925)
  line L156 (9.8225, -2.7484) -> (10.4374, -2.9482)
  line L157 (10.4374, -2.9482) -> (10.891, -3.6944)
  line L158 (10.891, -3.6944) -> (10.7054, -4.2654)
  line L159 (10.7054, -4.2654) -> (9.7685, -3.9609)
  line L160 (9.7685, -3.9609) -> (9.5001, -3.2425)
  line L161 (9.5001, -3.2425) -> (9.8225, -2.7484)
  line L162 (0.8202, -9.1077) -> (-1, -8.5)
  line L163 (-1, -8.5) -> (-1.357, -6.8189)
  line L164 (-1.357, -6.8189) -> (0, -6)
  line L165 (0, -6) -> (1.6404, -6.8063)
  line L166 (1.6404, -6.8063) -> (2, -8.5)
  line L167 (2, -8.5) -> (0.8202, -9.1077)
  line L168 (2.6736, 6.4706) -> (3.3781, 8.0522)
  line L169 (3.3781, 8.0522) -> (4.6898, 7.8504)
  line L170 (4.6898, 7.8504) -> (5.8052, 6.2889)
  line L171 (5.8052, 6.2889) -> (5.1059, 4.719)
  line L172 (5.1059, 4.719) -> (3.5267, 4.8541)
  line L173 (3.5267, 4.8541) -> (2.6736, 6.4706)
  line L174 (6.9801, -0.5432) -> (8.702, -0.7245)
  line L175 (8.702, -0.7245) -> (8.9154, -2.0344)
  line L176 (8.9154, -2.0344) -> (7.775, -3.5777)
  line L177 (7.775, -3.5777) -> (6.0658, -3.3977)
  line L178 (6.0658, -3.3977) -> (5.7063, -1.8541)
  line L179 (5.7063, -1.8541) -> (6.9801, -0.5432)
  line L180 (10.7785, -1.3057) -> (11.2993, -2.1887)
  line L181 (11.2993, -2.1887) -> (10.2999, -2.0834)
  line L182 (10.2999, -2.0834) -> (10.0348, -1.8876)
  line L183 (10.0348, -1.8876) -> (9.7957, -1.1372)
  line L184 (9.7957, -1.1372) -> (10.4141, -1.0365)
  line L185 (10.4141, -1.0365) -> (10.7785, -1.3057)
  line L186 (4.5725, 9.8475) -> (5.5732, 10.0699)
  line L187 (5.5732, 10.0699) -> (5.1643, 9.1519)
  line L188 (5.1643, 9.1519) -> (4.8961, 8.9604)
  line L189 (4.8961, 8.9604) -> (4.1086, 8.9648)
  line L190 (4.1086, 8.9648) -> (4.2039, 9.5842)
  line L191 (4.2039, 9.5842) -> (4.5725, 9.8475)
  line L192 (-7.9525, 7.3918) -> (-7.8548, 8.4122)
  line L193 (-7.8548, 8.4122) -> (-7.1081, 7.7396)
  line L194 (-7.1081, 7.7396) -> (-7.0089, 7.4254)
  line L195 (-7.0089, 7.4254) -> (-7.2564, 6.6778)
  line L196 (-7.2564, 6.6778) -> (-7.816, 6.9598)
  line L197 (-7.816, 6.9598) -> (-7.9525, 7.3918)
  line L198 (-9.4874, -5.2791) -> (-10.4278, -4.8709)
  line L199 (-10.4278, -4.8709) -> (-9.5574, -4.3686)
  line L200 (-9.5574, -4.3686) -> (-9.2278, -4.3712)
  line L201 (-9.2278, -4.3712) -> (-8.5933, -4.8377)
  line L202 (-8.5933, -4.8377) -> (-9.0344, -5.2828)
  line L203 (-9.0344, -5.2828) -> (-9.4874, -5.2791)
  line L204 (1.4101, -11.4226) -> (1.2014, -10.4396)
  line L205 (1.2014, -10.4396) -> (1.3057, -10.127)
  line L206 (1.3057, -10.127) -> (1.9455, -9.6677)
  line L207 (1.9455, -9.6677) -> (2.2324, -10.2247)
  line L208 (2.2324, -10.2247) -> (2.0889, -10.6544)
  line L209 (2.0889, -10.6544) -> (1.4101, -11.4226)
  line L210 (11.7371, -2.286) -> (12.0169, -2.7428)
  line L211 (12.0169, -2.7428) -> (11.4775, -2.4787)
  line L212 (11.4775, -2.4787) -> (11.5012, -2.2543)
  line L213 (11.5012, -2.2543) -> (11.7371, -2.286)
  line L214 (5.801, 10.4562) -> (6.322, 10.5812)
  line L215 (6.322, 10.5812) -> (5.9041, 10.1498)
  line L216 (5.9041, 10.1498) -> (5.698, 10.2417)
  line L217 (5.698, 10.2417) -> (5.801, 10.4562)
  line L218 (-8.1518, 8.7483) -> (-8.1097, 9.2824)
  line L219 (-8.1097, 9.2824) -> (-7.8286, 8.7516)
  line L220 (-7.8286, 8.7516) -> (-7.9796, 8.584)
  line L221 (-7.9796, 8.584) -> (-8.1518, 8.7483)
  line L222 (-10.8391, -5.0495) -> (-11.3341, -4.8444)
  line L223 (-11.3341, -4.8444) -> (-10.7425, -4.741)
  line L224 (-10.7425, -4.741) -> (-10.6297, -4.9365)
  line L225 (-10.6297, -4.9365) -> (-10.8391, -5.0495)
  line L226 (1.1049, -12.2764) -> (1.1894, -11.6818)
  line L227 (1.1894, -11.6818) -> (1.4101, -11.6349)
  line L228 (1.4101, -11.6349) -> (1.4529, -11.869)
  line L229 (1.4529, -11.869) -> (1.1049, -12.2764)
  circle A1 centre (0, 0) radius 19
  circle A2 centre (0, 0) radius 16
  circle A3 centre (0, 0) radius 4
  line L230 (1.6404, -3.6482) -> (7.5439, -14.1099)
  line L231 (3.2271, -2.3635) -> (10.0233, -12.4713)
  line L232 (3.245, 2.3388) -> (14.9583, 5.6788)
  line L233 (3.9765, 0.4327) -> (15.7505, 2.8145)
  line L234 (-1.2215, 3.8089) -> (-0.7785, 15.981)
  line L235 (0.8173, 3.9156) -> (2.1904, 15.8494)
  line L236 (-4, 0.0153) -> (-15.4395, 4.198)
  line L237 (-3.4714, 1.9873) -> (-14.3967, 6.981)
  line L238 (-1.2506, -3.7995) -> (-8.7636, -13.3865)
  line L239 (-2.9627, -2.6874) -> (-11.0881, -11.5349)
  dimension "d41" = 3
  dimension "d42" = 8
  dimension "d44" = 360
  constraint concentric A0 A2
  constraint concentric A0 A3
  constraint coincident A3 L230.start
  constraint coincident A2 L230.end
  constraint coincident A3 L231.start
  constraint coincident A2 L231.end
  measures "d41" distance of A1 A2
  measures "d42" diameter of A3
extrude "Extrude11" cut sketch "Sketch9" against normal blind 15 contours A2 A3 L232 L233 | A2 A3 L230 L231 | A2 A3 L234 L235 | A2 A3 L238 L239 | A2 A3 L236 L237
fillet "Fillet3" radius 3.5 1 edges at (-10.0233, 12.4713, -3.5)
fillet "Fillet4" radius 3.5 4 edges at (-14.9583, -5.6788, -3.5) (0.7785, -15.981, -3.5) (15.4395, -4.198, -3.5) (8.7636, 13.3865, -3.5)